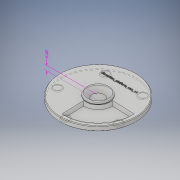
# Autodesk Inventor part: dissection_platform_v01
Saved by Autodesk Inventor 2019 (Build 230136000, 136)
## iProperties
Created: 2018-12-14
Part Number: dissection_platform_v01
Material: Generic
Document SubType Name: Modeling
Designer: Wilson Lab
Density: 1 g/cm^3
Appearance: Default
Author: Wilson Lab
Autodesk Inventor part; units mm, degrees
ref_plane "YZ Plane" through (0, 0, 0) normal (1, 0, 0) x (0, 1, 0)
ref_plane "XZ Plane" through (0, 0, 0) normal (0, 1, 0) x (-1, 0, 0)
ref_plane "XY Plane" through (0, 0, 0) normal (0, 0, 1) x (1, 0, 0)
sketch "Base Material Sketch" plane through (0, 0, 0) normal (0, 1, 0) x (-1, 0, 0)
  circle A0 centre (0, 0) radius 32.5
  dimension "d0" = 65
  constraints: 1 centre point, 1 coincident
  measures "d0" diameter of A0
extrude "Base Material Extrusion" add sketch "Base Material Sketch" along normal blind 4
sketch "Magnet Recess" plane through (0, 0, 0) normal (0, -1, 0) x (1, 0, 0)
  circle A0 centre (0, 0) radius 32.5 projected
  circle A1 centre (0, 27.5) radius 3.25
  line L0 (0, 0) -> (0, 32.5) construction
  circle A2 centre (0, 0) radius 32.5 construction
  circle A3 centre (-26.1541, 8.498) radius 3.25
  circle A4 centre (-16.1641, -22.248) radius 3.25
  circle A5 centre (16.1641, -22.248) radius 3.25
  circle A6 centre (26.1541, 8.498) radius 3.25
  dimension "d3" = 6.5
  dimension "d4" = 5
  dimension "d7" = 360
  constraints: 5 centre point, 2 end point, 1 point on line, 1 vertical, 1 vertical alignment, 12 other
  measures "d3" diameter of A1
  measures "d4" distance of A1.centre L0.end
extrude "Bottom Magnet Recess" cut sketch "Magnet Recess" against normal blind 1 contours A1 | A3 | A4 | A5 | A6
sketch "Central Well" plane through (0, 4, 0) normal (0, 1, 0) x (1, 0, 0)
  circle A0 centre (0, 0) radius 32.5 construction
  circle A1 centre (0, 0) radius 5
  dimension "d12" = 10
  constraints: 1 centre point, 1 coincident
  measures "d12" diameter of A1
extrude "Well Recess" cut sketch "Central Well" against normal blind 2
sketch "Sketch6" plane through (0, 4, 0) normal (0, 1, 0) x (1, 0, 0)
  circle A0 centre (0, 0) radius 9
  circle A1 centre (0, 0) radius 10
  dimension "d22" = 18
  dimension "d23" = 20
  constraints: 2 centre point, 2 coincident
  measures "d22" diameter of A0
  measures "d23" diameter of A1
extrude "Well Wall" add sketch "Sketch6" along normal blind 2
sketch "kimwipe recess sketch" plane through (0, 4, 0) normal (0, 1, 0) x (1, 0, 0)
  circle A0 centre (0, 0) radius 32.5 construction
  circle A1 centre (0, 0) radius 10 construction
  circle A2 centre (0, 0) radius 5 construction
  arc A3 (0, -12.5) -> (12.5, 0) centre (0, 0) ccw
  circle A4 centre (0, 0) radius 32.5 construction
  line L0 (0, 0) -> (-27.5, 0) construction
  line L1 (0, 0) -> (27.5, 0) construction
  line L2 (0, 0) -> (0, -27.5) construction
  line L3 (12.5, 0) -> (27.495, -0.5236)
  line L4 (0, -12.5) -> (0.5236, -27.495)
  arc A5 (0.5236, -27.495) -> (27.495, -0.5236) centre (0, 0) ccw
  dimension "d31" = 2.5
  dimension "d34" = 2
  dimension "d35" = 2
  dimension "d36" = 27.5
  constraints: 10 end point, 4 point on circle, 3 coincident, 2 centre point, 2 horizontal, 2 point on line, 1 perpendicular
  measures "d31" radial gap between concentric circles of A3 A1
  measures "d34" angle of L1 L3
  measures "d35" angle of L4 L2
  measures "d36" radius of A5
chamfer "Well Chamfer" distance 2 angle 45 2 edges at (-5, 4, 0) (-9, 4, 0)
fillet "Well Wall Fillet" radius 2 1 edges at (-10, 6, 0)
extrude "kimwipe recess" cut sketch "kimwipe recess sketch" against normal blind 2
chamfer "Kimwipe recess chamfer" distance 2 angle 45 4 edges at (0.2618, 4, 19.9975) (8.8388, 4, 8.8388) (19.9975, 4, 0.2618) (19.4454, 4, 19.4454)
fillet "Aesthetic Filet" radius 0.5 7 edges at (12.9141, 0, -22.248) (-19.4141, 0, -22.248) (-29.4041, 0, 8.498) (-3.25, 0, 27.5) (22.9041, 0, 8.498) (32.5, 0, 0) (32.5, 4, 0)
sketch "Sketch8" plane through (0, 4, 0) normal (0, 1, 0) x (1, 0, 0)
  line L0 (-6.854, 19.3116) -> (6.854, 19.3116) construction
  line L1 (6.854, 19.3116) -> (6.854, 17.5) construction
  line L2 (6.854, 17.5) -> (-6.854, 17.5) construction
  line L3 (-6.854, 17.5) -> (-6.854, 19.3116) construction
  circle A0 centre (0, 0) radius 17.5
  line L4 (-6.854, 17.5) -> (6.854, 17.5)
  line L5 (0, 0) -> (0, 17.5)
  line L6 (-14.128, 17.7085) -> (-14.3555, 17.7085)
  line L7 (-14.3555, 17.7085) -> (-14.3555, 17.8457)
  spline S0 degree 2 poles (-14.3555, 17.8457) (-14.408, 17.8019) (-14.4853, 17.7436) (-14.5378, 17.7188) knots 0 0 0 1 2 2 2
  spline S1 degree 2 poles (-14.5378, 17.7188) (-14.586, 17.6954) (-14.6895, 17.6706) (-14.7581, 17.6706) knots 0 0 0 1 2 2 2
  spline S2 degree 2 poles (-14.7581, 17.6706) (-14.869, 17.6706) (-15.0557, 17.7625) (-15.1213, 17.8515) knots 0 0 0 1 2 2 2
  spline S3 degree 2 poles (-15.1213, 17.8515) (-15.187, 17.9405) (-15.2599, 18.203) (-15.2599, 18.3737) knots 0 0 0 1 2 2 2
  spline S4 degree 2 poles (-15.2599, 18.3737) (-15.2599, 18.5517) (-15.168, 18.8113) (-15.0878, 18.909) knots 0 0 0 1 2 2 2
  spline S5 degree 2 poles (-15.0878, 18.909) (-15.0134, 18.9966) (-14.8048, 19.0972) (-14.6895, 19.0972) knots 0 0 0 1 2 2 2
  spline S6 degree 2 poles (-14.6895, 19.0972) (-14.5889, 19.0972) (-14.4387, 19.052) (-14.3555, 19.0053) knots 0 0 0 1 2 2 2
  line L8 (-14.3555, 19.0053) -> (-14.3555, 19.5888)
  line L9 (-14.3555, 19.5888) -> (-14.128, 19.5888)
  line L10 (-14.128, 19.5888) -> (-14.128, 17.7085)
  line L11 (-14.3555, 18.0368) -> (-14.3555, 18.8171)
  spline S7 degree 2 poles (-14.3555, 18.8171) (-14.4401, 18.858) (-14.5743, 18.8886) (-14.6516, 18.8886) knots 0 0 0 1 2 2 2
  spline S8 degree 2 poles (-14.6516, 18.8886) (-14.8267, 18.8886) (-15.025, 18.6261) (-15.025, 18.3781) knots 0 0 0 1 2 2 2
  spline S9 degree 2 poles (-15.025, 18.3781) (-15.025, 18.1389) (-14.8733, 17.8865) (-14.7056, 17.8865) knots 0 0 0 1 2 2 2
  spline S10 degree 2 poles (-14.7056, 17.8865) (-14.6166, 17.8865) (-14.4357, 17.9682) (-14.3555, 18.0368) knots 0 0 0 1 2 2 2
  line L12 (-13.5664, 17.7085) -> (-13.7939, 17.7085)
  line L13 (-13.7939, 17.7085) -> (-13.7939, 19.0593)
  line L14 (-13.7939, 19.0593) -> (-13.5664, 19.0593)
  line L15 (-13.5664, 19.0593) -> (-13.5664, 17.7085)
  line L16 (-13.5503, 19.2839) -> (-13.8085, 19.2839)
  line L17 (-13.8085, 19.2839) -> (-13.8085, 19.5202)
  line L18 (-13.8085, 19.5202) -> (-13.5503, 19.5202)
  line L19 (-13.5503, 19.5202) -> (-13.5503, 19.2839)
  spline S11 degree 2 poles (-12.8677, 17.6765) (-13.0033, 17.6765) (-13.2382, 17.7494) (-13.3155, 17.7902) knots 0 0 0 1 2 2 2
  line L20 (-13.3155, 17.7902) -> (-13.3155, 18.0455)
  line L21 (-13.3155, 18.0455) -> (-13.3038, 18.0455)
  spline S12 degree 2 poles (-13.3038, 18.0455) (-13.2746, 18.0222) (-13.1959, 17.9667) (-13.1302, 17.9361) knots 0 0 0 1 2 2 2
  spline S13 degree 2 poles (-13.1302, 17.9361) (-13.0733, 17.9084) (-12.9333, 17.8675) (-12.8589, 17.8675) knots 0 0 0 1 2 2 2
  spline S14 degree 2 poles (-12.8589, 17.8675) (-12.8049, 17.8675) (-12.681, 17.8923) (-12.6518, 17.9128) knots 0 0 0 1 2 2 2
  spline S15 degree 2 poles (-12.6518, 17.9128) (-12.6095, 17.9405) (-12.5716, 18.0032) (-12.5716, 18.0674) knots 0 0 0 1 2 2 2
  spline S16 degree 2 poles (-12.5716, 18.0674) (-12.5716, 18.1476) (-12.6591, 18.2308) (-12.7714, 18.2585) knots 0 0 0 1 2 2 2
  spline S17 degree 2 poles (-12.7714, 18.2585) (-12.8152, 18.2687) (-12.9552, 18.2979) (-13.015, 18.3139) knots 0 0 0 1 2 2 2
  spline S18 degree 2 poles (-13.015, 18.3139) (-13.1696, 18.3591) (-13.3096, 18.5458) (-13.3096, 18.6786) knots 0 0 0 1 2 2 2
  spline S19 degree 2 poles (-13.3096, 18.6786) (-13.3096, 18.8624) (-13.034, 19.0914) (-12.8064, 19.0914) knots 0 0 0 1 2 2 2
  spline S20 degree 2 poles (-12.8064, 19.0914) (-12.6941, 19.0914) (-12.4665, 19.0359) (-12.3892, 18.9936) knots 0 0 0 1 2 2 2
  line L22 (-12.3892, 18.9936) -> (-12.3892, 18.75)
  line L23 (-12.3892, 18.75) -> (-12.4009, 18.75)
  spline S21 degree 2 poles (-12.4009, 18.75) (-12.4884, 18.8201) (-12.7014, 18.9003) (-12.8108, 18.9003) knots 0 0 0 1 2 2 2
  spline S22 degree 2 poles (-12.8108, 18.9003) (-12.9231, 18.9003) (-13.0777, 18.8055) (-13.0777, 18.7107) knots 0 0 0 1 2 2 2
  spline S23 degree 2 poles (-13.0777, 18.7107) (-13.0777, 18.6246) (-12.9858, 18.5415) (-12.8837, 18.5152) knots 0 0 0 1 2 2 2
  spline S24 degree 2 poles (-12.8837, 18.5152) (-12.8341, 18.5021) (-12.7087, 18.4758) (-12.6401, 18.4598) knots 0 0 0 1 2 2 2
  spline S25 degree 2 poles (-12.6401, 18.4598) (-12.4913, 18.4218) (-12.3396, 18.2483) (-12.3396, 18.098) knots 0 0 0 1 2 2 2
  spline S26 degree 2 poles (-12.3396, 18.098) (-12.3396, 18.0105) (-12.4082, 17.8559) (-12.4753, 17.799) knots 0 0 0 1 2 2 2
  spline S27 degree 2 poles (-12.4753, 17.799) (-12.5468, 17.7392) (-12.7291, 17.6765) (-12.8677, 17.6765) knots 0 0 0 1 2 2 2
  spline S28 degree 2 poles (-11.7635, 17.6765) (-11.8991, 17.6765) (-12.134, 17.7494) (-12.2113, 17.7902) knots 0 0 0 1 2 2 2
  line L24 (-12.2113, 17.7902) -> (-12.2113, 18.0455)
  line L25 (-12.2113, 18.0455) -> (-12.1996, 18.0455)
  spline S29 degree 2 poles (-12.1996, 18.0455) (-12.1704, 18.0222) (-12.0917, 17.9667) (-12.026, 17.9361) knots 0 0 0 1 2 2 2
  spline S30 degree 2 poles (-12.026, 17.9361) (-11.9691, 17.9084) (-11.8291, 17.8675) (-11.7547, 17.8675) knots 0 0 0 1 2 2 2
  spline S31 degree 2 poles (-11.7547, 17.8675) (-11.7007, 17.8675) (-11.5767, 17.8923) (-11.5476, 17.9128) knots 0 0 0 1 2 2 2
  spline S32 degree 2 poles (-11.5476, 17.9128) (-11.5053, 17.9405) (-11.4673, 18.0032) (-11.4673, 18.0674) knots 0 0 0 1 2 2 2
  spline S33 degree 2 poles (-11.4673, 18.0674) (-11.4673, 18.1476) (-11.5549, 18.2308) (-11.6672, 18.2585) knots 0 0 0 1 2 2 2
  spline S34 degree 2 poles (-11.6672, 18.2585) (-11.7109, 18.2687) (-11.851, 18.2979) (-11.9108, 18.3139) knots 0 0 0 1 2 2 2
  spline S35 degree 2 poles (-11.9108, 18.3139) (-12.0654, 18.3591) (-12.2054, 18.5458) (-12.2054, 18.6786) knots 0 0 0 1 2 2 2
  spline S36 degree 2 poles (-12.2054, 18.6786) (-12.2054, 18.8624) (-11.9297, 19.0914) (-11.7022, 19.0914) knots 0 0 0 1 2 2 2
  spline S37 degree 2 poles (-11.7022, 19.0914) (-11.5899, 19.0914) (-11.3623, 19.0359) (-11.285, 18.9936) knots 0 0 0 1 2 2 2
  line L26 (-11.285, 18.9936) -> (-11.285, 18.75)
  line L27 (-11.285, 18.75) -> (-11.2967, 18.75)
  spline S38 degree 2 poles (-11.2967, 18.75) (-11.3842, 18.8201) (-11.5972, 18.9003) (-11.7066, 18.9003) knots 0 0 0 1 2 2 2
  spline S39 degree 2 poles (-11.7066, 18.9003) (-11.8189, 18.9003) (-11.9735, 18.8055) (-11.9735, 18.7107) knots 0 0 0 1 2 2 2
  spline S40 degree 2 poles (-11.9735, 18.7107) (-11.9735, 18.6246) (-11.8816, 18.5415) (-11.7795, 18.5152) knots 0 0 0 1 2 2 2
  spline S41 degree 2 poles (-11.7795, 18.5152) (-11.7299, 18.5021) (-11.6045, 18.4758) (-11.5359, 18.4598) knots 0 0 0 1 2 2 2
  spline S42 degree 2 poles (-11.5359, 18.4598) (-11.3871, 18.4218) (-11.2354, 18.2483) (-11.2354, 18.098) knots 0 0 0 1 2 2 2
  spline S43 degree 2 poles (-11.2354, 18.098) (-11.2354, 18.0105) (-11.304, 17.8559) (-11.3711, 17.799) knots 0 0 0 1 2 2 2
  spline S44 degree 2 poles (-11.3711, 17.799) (-11.4425, 17.7392) (-11.6249, 17.6765) (-11.7635, 17.6765) knots 0 0 0 1 2 2 2
  spline S45 degree 2 poles (-10.4375, 17.6779) (-10.7613, 17.6779) (-11.1173, 18.0411) (-11.1173, 18.3766) knots 0 0 0 1 2 2 2
  spline S46 degree 2 poles (-11.1173, 18.3766) (-11.1173, 18.7063) (-10.7716, 19.0972) (-10.4929, 19.0972) knots 0 0 0 1 2 2 2
  spline S47 degree 2 poles (-10.4929, 19.0972) (-10.3675, 19.0972) (-10.1735, 19.0243) (-10.102, 18.947) knots 0 0 0 1 2 2 2
  spline S48 degree 2 poles (-10.102, 18.947) (-10.0291, 18.8697) (-9.9518, 18.6465) (-9.9518, 18.4846) knots 0 0 0 1 2 2 2
  line L28 (-9.9518, 18.4846) -> (-9.9518, 18.3606)
  line L29 (-9.9518, 18.3606) -> (-10.8868, 18.3606)
  spline S49 degree 2 poles (-10.8868, 18.3606) (-10.8868, 18.1257) (-10.6505, 17.8763) (-10.4404, 17.8763) knots 0 0 0 1 2 2 2
  spline S50 degree 2 poles (-10.4404, 17.8763) (-10.366, 17.8763) (-10.2216, 17.9098) (-10.1633, 17.9361) knots 0 0 0 1 2 2 2
  spline S51 degree 2 poles (-10.1633, 17.9361) (-10.102, 17.9653) (-10.0174, 18.0163) (-9.9897, 18.0397) knots 0 0 0 1 2 2 2
  line L30 (-9.9897, 18.0397) -> (-9.9766, 18.0397)
  line L31 (-9.9766, 18.0397) -> (-9.9766, 17.7917)
  spline S52 degree 2 poles (-9.9766, 17.7917) (-10.016, 17.7756) (-10.1356, 17.729) (-10.1823, 17.7158) knots 0 0 0 1 2 2 2
  spline S53 degree 2 poles (-10.1823, 17.7158) (-10.2479, 17.6969) (-10.3558, 17.6779) (-10.4375, 17.6779) knots 0 0 0 1 2 2 2
  spline S54 degree 2 poles (-10.1735, 18.5342) (-10.1764, 18.6261) (-10.2143, 18.7603) (-10.2508, 18.8055) knots 0 0 0 1 2 2 2
  spline S55 degree 2 poles (-10.2508, 18.8055) (-10.2902, 18.8565) (-10.4142, 18.9105) (-10.5061, 18.9105) knots 0 0 0 1 2 2 2
  spline S56 degree 2 poles (-10.5061, 18.9105) (-10.5965, 18.9105) (-10.7234, 18.8565) (-10.7759, 18.804) knots 0 0 0 1 2 2 2
  spline S57 degree 2 poles (-10.7759, 18.804) (-10.827, 18.75) (-10.8795, 18.6202) (-10.8868, 18.5342) knots 0 0 0 1 2 2 2
  line L32 (-10.8868, 18.5342) -> (-10.1735, 18.5342)
  spline S58 degree 2 poles (-9.1845, 17.6779) (-9.3246, 17.6779) (-9.5565, 17.764) (-9.6396, 17.8515) knots 0 0 0 1 2 2 2
  spline S59 degree 2 poles (-9.6396, 17.8515) (-9.7228, 17.9376) (-9.8147, 18.203) (-9.8147, 18.381) knots 0 0 0 1 2 2 2
  spline S60 degree 2 poles (-9.8147, 18.381) (-9.8147, 18.559) (-9.7199, 18.8186) (-9.6396, 18.9061) knots 0 0 0 1 2 2 2
  spline S61 degree 2 poles (-9.6396, 18.9061) (-9.5594, 18.9951) (-9.3216, 19.0899) (-9.1845, 19.0899) knots 0 0 0 1 2 2 2
  spline S62 degree 2 poles (-9.1845, 19.0899) (-9.0737, 19.0899) (-8.8665, 19.0272) (-8.7863, 18.9863) knots 0 0 0 1 2 2 2
  line L33 (-8.7863, 18.9863) -> (-8.7863, 18.7311)
  line L34 (-8.7863, 18.7311) -> (-8.7994, 18.7311)
  spline S63 degree 2 poles (-8.7994, 18.7311) (-8.8242, 18.7515) (-8.9001, 18.804) (-8.9541, 18.8317) knots 0 0 0 1 2 2 2
  spline S64 degree 2 poles (-8.9541, 18.8317) (-9.0022, 18.8551) (-9.1306, 18.8915) (-9.1889, 18.8915) knots 0 0 0 1 2 2 2
  spline S65 degree 2 poles (-9.1889, 18.8915) (-9.3654, 18.8915) (-9.5798, 18.6246) (-9.5798, 18.381) knots 0 0 0 1 2 2 2
  spline S66 degree 2 poles (-9.5798, 18.381) (-9.5798, 18.1432) (-9.3727, 17.8763) (-9.1889, 17.8763) knots 0 0 0 1 2 2 2
  spline S67 degree 2 poles (-9.1889, 17.8763) (-9.078, 17.8763) (-8.8767, 17.9682) (-8.7994, 18.0397) knots 0 0 0 1 2 2 2
  line L35 (-8.7994, 18.0397) -> (-8.7863, 18.0397)
  line L36 (-8.7863, 18.0397) -> (-8.7863, 17.7844)
  spline S68 degree 2 poles (-8.7863, 17.7844) (-8.8199, 17.7684) (-8.922, 17.7231) (-8.9628, 17.7129) knots 0 0 0 1 2 2 2
  spline S69 degree 2 poles (-8.9628, 17.7129) (-9.0212, 17.6954) (-9.113, 17.6779) (-9.1845, 17.6779) knots 0 0 0 1 2 2 2
  spline S70 degree 2 poles (-8.1707, 17.6823) (-8.356, 17.6823) (-8.5646, 17.8938) (-8.5646, 18.1228) knots 0 0 0 1 2 2 2
  line L37 (-8.5646, 18.1228) -> (-8.5646, 18.8711)
  line L38 (-8.5646, 18.8711) -> (-8.7177, 18.8711)
  line L39 (-8.7177, 18.8711) -> (-8.7177, 19.0593)
  line L40 (-8.7177, 19.0593) -> (-8.5646, 19.0593)
  line L41 (-8.5646, 19.0593) -> (-8.5646, 19.4473)
  line L42 (-8.5646, 19.4473) -> (-8.337, 19.4473)
  line L43 (-8.337, 19.4473) -> (-8.337, 19.0593)
  line L44 (-8.337, 19.0593) -> (-7.9184, 19.0593)
  line L45 (-7.9184, 19.0593) -> (-7.9184, 18.8711)
  line L46 (-7.9184, 18.8711) -> (-8.337, 18.8711)
  line L47 (-8.337, 18.8711) -> (-8.337, 18.2278)
  spline S71 degree 2 poles (-8.337, 18.2278) (-8.337, 18.1257) (-8.3297, 18.0134) (-8.3049, 17.9653) knots 0 0 0 1 2 2 2
  spline S72 degree 2 poles (-8.3049, 17.9653) (-8.2845, 17.923) (-8.1926, 17.8807) (-8.1139, 17.8807) knots 0 0 0 1 2 2 2
  spline S73 degree 2 poles (-8.1139, 17.8807) (-8.0584, 17.8807) (-7.9549, 17.9142) (-7.9315, 17.9244) knots 0 0 0 1 2 2 2
  line L48 (-7.9315, 17.9244) -> (-7.9184, 17.9244)
  line L49 (-7.9184, 17.9244) -> (-7.9184, 17.7202)
  spline S74 degree 2 poles (-7.9184, 17.7202) (-7.9826, 17.7027) (-8.1139, 17.6823) (-8.1707, 17.6823) knots 0 0 0 1 2 2 2
  line L50 (-7.5187, 17.7085) -> (-7.7463, 17.7085)
  line L51 (-7.7463, 17.7085) -> (-7.7463, 19.0593)
  line L52 (-7.7463, 19.0593) -> (-7.5187, 19.0593)
  line L53 (-7.5187, 19.0593) -> (-7.5187, 17.7085)
  line L54 (-7.5027, 19.2839) -> (-7.7609, 19.2839)
  line L55 (-7.7609, 19.2839) -> (-7.7609, 19.5202)
  line L56 (-7.7609, 19.5202) -> (-7.5027, 19.5202)
  line L57 (-7.5027, 19.5202) -> (-7.5027, 19.2839)
  spline S75 degree 2 poles (-6.0746, 18.3839) (-6.0746, 18.0426) (-6.4028, 17.6706) (-6.6771, 17.6706) knots 0 0 0 1 2 2 2
  spline S76 degree 2 poles (-6.6771, 17.6706) (-6.9586, 17.6706) (-7.281, 18.0543) (-7.281, 18.3839) knots 0 0 0 1 2 2 2
  spline S77 degree 2 poles (-7.281, 18.3839) (-7.281, 18.7223) (-6.9484, 19.0972) (-6.6771, 19.0972) knots 0 0 0 1 2 2 2
  spline S78 degree 2 poles (-6.6771, 19.0972) (-6.4028, 19.0972) (-6.0746, 18.7238) (-6.0746, 18.3839) knots 0 0 0 1 2 2 2
  spline S79 degree 2 poles (-6.3095, 18.3839) (-6.3095, 18.6465) (-6.5006, 18.9017) (-6.6771, 18.9017) knots 0 0 0 1 2 2 2
  spline S80 degree 2 poles (-6.6771, 18.9017) (-6.8536, 18.9017) (-7.0461, 18.6465) (-7.0461, 18.3839) knots 0 0 0 1 2 2 2
  spline S81 degree 2 poles (-7.0461, 18.3839) (-7.0461, 18.1286) (-6.8536, 17.8661) (-6.6771, 17.8661) knots 0 0 0 1 2 2 2
  spline S82 degree 2 poles (-6.6771, 17.8661) (-6.502, 17.8661) (-6.3095, 18.1243) (-6.3095, 18.3839) knots 0 0 0 1 2 2 2
  line L58 (-4.7808, 17.7085) -> (-5.0083, 17.7085)
  line L59 (-5.0083, 17.7085) -> (-5.0083, 18.4787)
  spline S83 degree 2 poles (-5.0083, 18.4787) (-5.0083, 18.5721) (-5.0259, 18.7325) (-5.0521, 18.7807) knots 0 0 0 1 2 2 2
  spline S84 degree 2 poles (-5.0521, 18.7807) (-5.0798, 18.8317) (-5.179, 18.8813) (-5.2636, 18.8813) knots 0 0 0 1 2 2 2
  spline S85 degree 2 poles (-5.2636, 18.8813) (-5.3482, 18.8813) (-5.5276, 18.7909) (-5.6137, 18.718) knots 0 0 0 1 2 2 2
  line L60 (-5.6137, 18.718) -> (-5.6137, 17.7085)
  line L61 (-5.6137, 17.7085) -> (-5.8412, 17.7085)
  line L62 (-5.8412, 17.7085) -> (-5.8412, 19.0593)
  line L63 (-5.8412, 19.0593) -> (-5.6137, 19.0593)
  line L64 (-5.6137, 19.0593) -> (-5.6137, 18.909)
  spline S86 degree 2 poles (-5.6137, 18.909) (-5.5116, 19.0009) (-5.3147, 19.0972) (-5.2038, 19.0972) knots 0 0 0 1 2 2 2
  spline S87 degree 2 poles (-5.2038, 19.0972) (-5.0054, 19.0972) (-4.7808, 18.8346) (-4.7808, 18.5852) knots 0 0 0 1 2 2 2
  line L65 (-4.7808, 18.5852) -> (-4.7808, 17.7085)
  line L66 (-3.2565, 17.3468) -> (-4.6451, 17.3468)
  line L67 (-4.6451, 17.3468) -> (-4.6451, 17.5029)
  line L68 (-4.6451, 17.5029) -> (-3.2565, 17.5029)
  line L69 (-3.2565, 17.5029) -> (-3.2565, 17.3468)
  spline S88 degree 2 poles (-1.9787, 18.4204) (-1.9787, 18.082) (-2.3011, 17.6823) (-2.5476, 17.6823) knots 0 0 0 1 2 2 2
  spline S89 degree 2 poles (-2.5476, 17.6823) (-2.6482, 17.6823) (-2.8028, 17.729) (-2.8831, 17.7771) knots 0 0 0 1 2 2 2
  line L70 (-2.8831, 17.7771) -> (-2.8831, 17.2111)
  line L71 (-2.8831, 17.2111) -> (-3.1106, 17.2111)
  line L72 (-3.1106, 17.2111) -> (-3.1106, 19.0593)
  line L73 (-3.1106, 19.0593) -> (-2.8831, 19.0593)
  line L74 (-2.8831, 19.0593) -> (-2.8831, 18.9178)
  spline S90 degree 2 poles (-2.8831, 18.9178) (-2.7985, 18.9951) (-2.5913, 19.0972) (-2.4703, 19.0972) knots 0 0 0 1 2 2 2
  spline S91 degree 2 poles (-2.4703, 19.0972) (-2.2383, 19.0972) (-1.9787, 18.7296) (-1.9787, 18.4204) knots 0 0 0 1 2 2 2
  spline S92 degree 2 poles (-2.2135, 18.3941) (-2.2135, 18.6261) (-2.3609, 18.8813) (-2.5257, 18.8813) knots 0 0 0 1 2 2 2
  spline S93 degree 2 poles (-2.5257, 18.8813) (-2.622, 18.8813) (-2.8028, 18.7953) (-2.8831, 18.7282) knots 0 0 0 1 2 2 2
  line L75 (-2.8831, 18.7282) -> (-2.8831, 17.9609)
  spline S94 degree 2 poles (-2.8831, 17.9609) (-2.7941, 17.9186) (-2.6672, 17.8865) (-2.5855, 17.8865) knots 0 0 0 1 2 2 2
  spline S95 degree 2 poles (-2.5855, 17.8865) (-2.409, 17.8865) (-2.2135, 18.1462) (-2.2135, 18.3941) knots 0 0 0 1 2 2 2
  line L76 (-1.5105, 17.7085) -> (-1.738, 17.7085)
  line L77 (-1.738, 17.7085) -> (-1.738, 19.5888)
  line L78 (-1.738, 19.5888) -> (-1.5105, 19.5888)
  line L79 (-1.5105, 19.5888) -> (-1.5105, 17.7085)
  spline S96 degree 2 poles (-0.4237, 17.8515) (-0.4515, 17.8311) (-0.5448, 17.7581) (-0.5886, 17.7363) knots 0 0 0 1 2 2 2
  spline S97 degree 2 poles (-0.5886, 17.7363) (-0.6484, 17.7042) (-0.7607, 17.6706) (-0.8628, 17.6706) knots 0 0 0 1 2 2 2
  spline S98 degree 2 poles (-0.8628, 17.6706) (-0.9459, 17.6706) (-1.0962, 17.7333) (-1.1531, 17.7902) knots 0 0 0 1 2 2 2
  spline S99 degree 2 poles (-1.1531, 17.7902) (-1.207, 17.8457) (-1.2727, 18.009) (-1.2727, 18.0995) knots 0 0 0 1 2 2 2
  spline S100 degree 2 poles (-1.2727, 18.0995) (-1.2727, 18.2395) (-1.1545, 18.4379) (-1.0262, 18.4948) knots 0 0 0 1 2 2 2
  spline S101 degree 2 poles (-1.0262, 18.4948) (-0.9124, 18.5473) (-0.6032, 18.5867) (-0.4237, 18.5969) knots 0 0 0 1 2 2 2
  line L80 (-0.4237, 18.5969) -> (-0.4237, 18.6406)
  spline S102 degree 2 poles (-0.4237, 18.6406) (-0.4237, 18.7194) (-0.4719, 18.8171) (-0.5156, 18.8449) knots 0 0 0 1 2 2 2
  spline S103 degree 2 poles (-0.5156, 18.8449) (-0.5594, 18.8726) (-0.6848, 18.8901) (-0.7519, 18.8901) knots 0 0 0 1 2 2 2
  spline S104 degree 2 poles (-0.7519, 18.8901) (-0.8307, 18.8901) (-1.0437, 18.8434) (-1.1502, 18.7982) knots 0 0 0 1 2 2 2
  line L81 (-1.1502, 18.7982) -> (-1.1633, 18.7982)
  line L82 (-1.1633, 18.7982) -> (-1.1633, 19.0301)
  spline S105 degree 2 poles (-1.1633, 19.0301) (-1.1006, 19.0476) (-0.8657, 19.0914) (-0.7505, 19.0914) knots 0 0 0 1 2 2 2
  spline S106 degree 2 poles (-0.7505, 19.0914) (-0.6105, 19.0914) (-0.4194, 19.0476) (-0.3435, 18.9907) knots 0 0 0 1 2 2 2
  spline S107 degree 2 poles (-0.3435, 18.9907) (-0.2691, 18.9353) (-0.1962, 18.7588) (-0.1962, 18.6319) knots 0 0 0 1 2 2 2
  line L83 (-0.1962, 18.6319) -> (-0.1962, 17.7085)
  line L84 (-0.1962, 17.7085) -> (-0.4237, 17.7085)
  line L85 (-0.4237, 17.7085) -> (-0.4237, 17.8515)
  line L86 (-0.4237, 18.0411) -> (-0.4237, 18.416)
  spline S108 degree 2 poles (-0.4237, 18.416) (-0.5054, 18.4087) (-0.7519, 18.3839) (-0.8293, 18.3606) knots 0 0 0 1 2 2 2
  spline S109 degree 2 poles (-0.8293, 18.3606) (-0.9197, 18.3329) (-1.0378, 18.2176) (-1.0378, 18.1155) knots 0 0 0 1 2 2 2
  spline S110 degree 2 poles (-1.0378, 18.1155) (-1.0378, 17.9988) (-0.9066, 17.8807) (-0.7811, 17.8807) knots 0 0 0 1 2 2 2
  spline S111 degree 2 poles (-0.7811, 17.8807) (-0.6746, 17.8807) (-0.4996, 17.9726) (-0.4237, 18.0411) knots 0 0 0 1 2 2 2
  spline S112 degree 2 poles (0.5317, 17.6823) (0.3464, 17.6823) (0.1378, 17.8938) (0.1378, 18.1228) knots 0 0 0 1 2 2 2
  line L87 (0.1378, 18.1228) -> (0.1378, 18.8711)
  line L88 (0.1378, 18.8711) -> (-0.0153, 18.8711)
  line L89 (-0.0153, 18.8711) -> (-0.0153, 19.0593)
  line L90 (-0.0153, 19.0593) -> (0.1378, 19.0593)
  line L91 (0.1378, 19.0593) -> (0.1378, 19.4473)
  line L92 (0.1378, 19.4473) -> (0.3654, 19.4473)
  line L93 (0.3654, 19.4473) -> (0.3654, 19.0593)
  line L94 (0.3654, 19.0593) -> (0.784, 19.0593)
  line L95 (0.784, 19.0593) -> (0.784, 18.8711)
  line L96 (0.784, 18.8711) -> (0.3654, 18.8711)
  line L97 (0.3654, 18.8711) -> (0.3654, 18.2278)
  spline S113 degree 2 poles (0.3654, 18.2278) (0.3654, 18.1257) (0.3727, 18.0134) (0.3975, 17.9653) knots 0 0 0 1 2 2 2
  spline S114 degree 2 poles (0.3975, 17.9653) (0.4179, 17.923) (0.5098, 17.8807) (0.5886, 17.8807) knots 0 0 0 1 2 2 2
  spline S115 degree 2 poles (0.5886, 17.8807) (0.644, 17.8807) (0.7476, 17.9142) (0.7709, 17.9244) knots 0 0 0 1 2 2 2
  line L98 (0.7709, 17.9244) -> (0.784, 17.9244)
  line L99 (0.784, 17.9244) -> (0.784, 17.7202)
  spline S116 degree 2 poles (0.784, 17.7202) (0.7199, 17.7027) (0.5886, 17.6823) (0.5317, 17.6823) knots 0 0 0 1 2 2 2
  line L100 (1.6622, 19.37) -> (1.6505, 19.37)
  spline S117 degree 2 poles (1.6505, 19.37) (1.6199, 19.3816) (1.5061, 19.4021) (1.4609, 19.4021) knots 0 0 0 1 2 2 2
  spline S118 degree 2 poles (1.4609, 19.4021) (1.3179, 19.4021) (1.1954, 19.2737) (1.1954, 19.1045) knots 0 0 0 1 2 2 2
  line L101 (1.1954, 19.1045) -> (1.1954, 19.0593)
  line L102 (1.1954, 19.0593) -> (1.5717, 19.0593)
  line L103 (1.5717, 19.0593) -> (1.5717, 18.8711)
  line L104 (1.5717, 18.8711) -> (1.2027, 18.8711)
  line L105 (1.2027, 18.8711) -> (1.2027, 17.7085)
  line L106 (1.2027, 17.7085) -> (0.9751, 17.7085)
  line L107 (0.9751, 17.7085) -> (0.9751, 18.8711)
  line L108 (0.9751, 18.8711) -> (0.822, 18.8711)
  line L109 (0.822, 18.8711) -> (0.822, 19.0593)
  line L110 (0.822, 19.0593) -> (0.9751, 19.0593)
  line L111 (0.9751, 19.0593) -> (0.9751, 19.1045)
  spline S119 degree 2 poles (0.9751, 19.1045) (0.9751, 19.3466) (1.21, 19.6004) (1.4288, 19.6004) knots 0 0 0 1 2 2 2
  spline S120 degree 2 poles (1.4288, 19.6004) (1.4915, 19.6004) (1.6126, 19.5873) (1.6622, 19.5786) knots 0 0 0 1 2 2 2
  line L112 (1.6622, 19.5786) -> (1.6622, 19.37)
  spline S121 degree 2 poles (2.8495, 18.3839) (2.8495, 18.0426) (2.5213, 17.6706) (2.2471, 17.6706) knots 0 0 0 1 2 2 2
  spline S122 degree 2 poles (2.2471, 17.6706) (1.9656, 17.6706) (1.6432, 18.0543) (1.6432, 18.3839) knots 0 0 0 1 2 2 2
  spline S123 degree 2 poles (1.6432, 18.3839) (1.6432, 18.7223) (1.9758, 19.0972) (2.2471, 19.0972) knots 0 0 0 1 2 2 2
  spline S124 degree 2 poles (2.2471, 19.0972) (2.5213, 19.0972) (2.8495, 18.7238) (2.8495, 18.3839) knots 0 0 0 1 2 2 2
  spline S125 degree 2 poles (2.6147, 18.3839) (2.6147, 18.6465) (2.4236, 18.9017) (2.2471, 18.9017) knots 0 0 0 1 2 2 2
  spline S126 degree 2 poles (2.2471, 18.9017) (2.0706, 18.9017) (1.878, 18.6465) (1.878, 18.3839) knots 0 0 0 1 2 2 2
  spline S127 degree 2 poles (1.878, 18.3839) (1.878, 18.1286) (2.0706, 17.8661) (2.2471, 17.8661) knots 0 0 0 1 2 2 2
  spline S128 degree 2 poles (2.2471, 17.8661) (2.4221, 17.8661) (2.6147, 18.1243) (2.6147, 18.3839) knots 0 0 0 1 2 2 2
  line L113 (3.7991, 18.8157) -> (3.7874, 18.8157)
  spline S129 degree 2 poles (3.7874, 18.8157) (3.7612, 18.823) (3.7043, 18.8259) (3.6649, 18.8259) knots 0 0 0 1 2 2 2
  spline S130 degree 2 poles (3.6649, 18.8259) (3.573, 18.8259) (3.3921, 18.7457) (3.3105, 18.6669) knots 0 0 0 1 2 2 2
  line L114 (3.3105, 18.6669) -> (3.3105, 17.7085)
  line L115 (3.3105, 17.7085) -> (3.0829, 17.7085)
  line L116 (3.0829, 17.7085) -> (3.0829, 19.0593)
  line L117 (3.0829, 19.0593) -> (3.3105, 19.0593)
  line L118 (3.3105, 19.0593) -> (3.3105, 18.858)
  spline S131 degree 2 poles (3.3105, 18.858) (3.4344, 18.9688) (3.6197, 19.0593) (3.7072, 19.0593) knots 0 0 0 1 2 2 2
  spline S132 degree 2 poles (3.7072, 19.0593) (3.7422, 19.0593) (3.7772, 19.0564) (3.7991, 19.052) knots 0 0 0 1 2 2 2
  line L119 (3.7991, 19.052) -> (3.7991, 18.8157)
  line L120 (5.5072, 17.7085) -> (5.5072, 18.4904)
  spline S133 degree 2 poles (5.5072, 18.4904) (5.5072, 18.5838) (5.4926, 18.7427) (5.4693, 18.7865) knots 0 0 0 1 2 2 2
  spline S134 degree 2 poles (5.4693, 18.7865) (5.4459, 18.8346) (5.357, 18.8813) (5.2797, 18.8813) knots 0 0 0 1 2 2 2
  spline S135 degree 2 poles (5.2797, 18.8813) (5.2096, 18.8813) (5.0492, 18.7953) (4.9646, 18.7136) knots 0 0 0 1 2 2 2
  spline S136 degree 2 poles (4.9646, 18.7136) (4.966, 18.6932) (4.969, 18.6363) (4.969, 18.5983) knots 0 0 0 1 2 2 2
  line L121 (4.969, 18.5983) -> (4.969, 17.7085)
  line L122 (4.969, 17.7085) -> (4.7414, 17.7085)
  line L123 (4.7414, 17.7085) -> (4.7414, 18.4904)
  spline S137 degree 2 poles (4.7414, 18.4904) (4.7414, 18.5838) (4.7268, 18.7427) (4.7035, 18.7865) knots 0 0 0 1 2 2 2
  spline S138 degree 2 poles (4.7035, 18.7865) (4.6801, 18.8346) (4.5912, 18.8813) (4.5139, 18.8813) knots 0 0 0 1 2 2 2
  spline S139 degree 2 poles (4.5139, 18.8813) (4.4409, 18.8813) (4.279, 18.7894) (4.2032, 18.718) knots 0 0 0 1 2 2 2
  line L124 (4.2032, 18.718) -> (4.2032, 17.7085)
  line L125 (4.2032, 17.7085) -> (3.9756, 17.7085)
  line L126 (3.9756, 17.7085) -> (3.9756, 19.0593)
  line L127 (3.9756, 19.0593) -> (4.2032, 19.0593)
  line L128 (4.2032, 19.0593) -> (4.2032, 18.9105)
  spline S140 degree 2 poles (4.2032, 18.9105) (4.2921, 18.9995) (4.4672, 19.0972) (4.5722, 19.0972) knots 0 0 0 1 2 2 2
  spline S141 degree 2 poles (4.5722, 19.0972) (4.6918, 19.0972) (4.8771, 18.9878) (4.9252, 18.8638) knots 0 0 0 1 2 2 2
  spline S142 degree 2 poles (4.9252, 18.8638) (5.0288, 18.9791) (5.2242, 19.0972) (5.338, 19.0972) knots 0 0 0 1 2 2 2
  spline S143 degree 2 poles (5.338, 19.0972) (5.4255, 19.0972) (5.5685, 19.0432) (5.621, 18.982) knots 0 0 0 1 2 2 2
  spline S144 degree 2 poles (5.621, 18.982) (5.675, 18.9207) (5.7348, 18.7369) (5.7348, 18.5983) knots 0 0 0 1 2 2 2
  line L129 (5.7348, 18.5983) -> (5.7348, 17.7085)
  line L130 (5.7348, 17.7085) -> (5.5072, 17.7085)
  line L131 (7.2591, 17.3468) -> (5.8704, 17.3468)
  line L132 (5.8704, 17.3468) -> (5.8704, 17.5029)
  line L133 (5.8704, 17.5029) -> (7.2591, 17.5029)
  line L134 (7.2591, 17.5029) -> (7.2591, 17.3468)
  line L135 (8.9365, 17.7085) -> (8.9365, 18.4904)
  spline S145 degree 2 poles (8.9365, 18.4904) (8.9365, 18.5838) (8.922, 18.7427) (8.8986, 18.7865) knots 0 0 0 1 2 2 2
  spline S146 degree 2 poles (8.8986, 18.7865) (8.8753, 18.8346) (8.7863, 18.8813) (8.709, 18.8813) knots 0 0 0 1 2 2 2
  spline S147 degree 2 poles (8.709, 18.8813) (8.639, 18.8813) (8.4785, 18.7953) (8.3939, 18.7136) knots 0 0 0 1 2 2 2
  spline S148 degree 2 poles (8.3939, 18.7136) (8.3954, 18.6932) (8.3983, 18.6363) (8.3983, 18.5983) knots 0 0 0 1 2 2 2
  line L136 (8.3983, 18.5983) -> (8.3983, 17.7085)
  line L137 (8.3983, 17.7085) -> (8.1707, 17.7085)
  line L138 (8.1707, 17.7085) -> (8.1707, 18.4904)
  spline S149 degree 2 poles (8.1707, 18.4904) (8.1707, 18.5838) (8.1562, 18.7427) (8.1328, 18.7865) knots 0 0 0 1 2 2 2
  spline S150 degree 2 poles (8.1328, 18.7865) (8.1095, 18.8346) (8.0205, 18.8813) (7.9432, 18.8813) knots 0 0 0 1 2 2 2
  spline S151 degree 2 poles (7.9432, 18.8813) (7.8703, 18.8813) (7.7083, 18.7894) (7.6325, 18.718) knots 0 0 0 1 2 2 2
  line L139 (7.6325, 18.718) -> (7.6325, 17.7085)
  line L140 (7.6325, 17.7085) -> (7.4049, 17.7085)
  line L141 (7.4049, 17.7085) -> (7.4049, 19.0593)
  line L142 (7.4049, 19.0593) -> (7.6325, 19.0593)
  line L143 (7.6325, 19.0593) -> (7.6325, 18.9105)
  spline S152 degree 2 poles (7.6325, 18.9105) (7.7215, 18.9995) (7.8965, 19.0972) (8.0015, 19.0972) knots 0 0 0 1 2 2 2
  spline S153 degree 2 poles (8.0015, 19.0972) (8.1212, 19.0972) (8.3064, 18.9878) (8.3545, 18.8638) knots 0 0 0 1 2 2 2
  spline S154 degree 2 poles (8.3545, 18.8638) (8.4581, 18.9791) (8.6536, 19.0972) (8.7673, 19.0972) knots 0 0 0 1 2 2 2
  spline S155 degree 2 poles (8.7673, 19.0972) (8.8549, 19.0972) (8.9978, 19.0432) (9.0503, 18.982) knots 0 0 0 1 2 2 2
  spline S156 degree 2 poles (9.0503, 18.982) (9.1043, 18.9207) (9.1641, 18.7369) (9.1641, 18.5983) knots 0 0 0 1 2 2 2
  line L144 (9.1641, 18.5983) -> (9.1641, 17.7085)
  line L145 (9.1641, 17.7085) -> (8.9365, 17.7085)
  line L146 (11.0152, 17.7085) -> (11.0152, 18.4904)
  spline S157 degree 2 poles (11.0152, 18.4904) (11.0152, 18.5838) (11.0006, 18.7427) (10.9772, 18.7865) knots 0 0 0 1 2 2 2
  spline S158 degree 2 poles (10.9772, 18.7865) (10.9539, 18.8346) (10.8649, 18.8813) (10.7876, 18.8813) knots 0 0 0 1 2 2 2
  spline S159 degree 2 poles (10.7876, 18.8813) (10.7176, 18.8813) (10.5571, 18.7953) (10.4725, 18.7136) knots 0 0 0 1 2 2 2
  spline S160 degree 2 poles (10.4725, 18.7136) (10.474, 18.6932) (10.4769, 18.6363) (10.4769, 18.5983) knots 0 0 0 1 2 2 2
  line L147 (10.4769, 18.5983) -> (10.4769, 17.7085)
  line L148 (10.4769, 17.7085) -> (10.2494, 17.7085)
  line L149 (10.2494, 17.7085) -> (10.2494, 18.4904)
  spline S161 degree 2 poles (10.2494, 18.4904) (10.2494, 18.5838) (10.2348, 18.7427) (10.2114, 18.7865) knots 0 0 0 1 2 2 2
  spline S162 degree 2 poles (10.2114, 18.7865) (10.1881, 18.8346) (10.0991, 18.8813) (10.0218, 18.8813) knots 0 0 0 1 2 2 2
  spline S163 degree 2 poles (10.0218, 18.8813) (9.9489, 18.8813) (9.787, 18.7894) (9.7111, 18.718) knots 0 0 0 1 2 2 2
  line L150 (9.7111, 18.718) -> (9.7111, 17.7085)
  line L151 (9.7111, 17.7085) -> (9.4836, 17.7085)
  line L152 (9.4836, 17.7085) -> (9.4836, 19.0593)
  line L153 (9.4836, 19.0593) -> (9.7111, 19.0593)
  line L154 (9.7111, 19.0593) -> (9.7111, 18.9105)
  spline S164 degree 2 poles (9.7111, 18.9105) (9.8001, 18.9995) (9.9751, 19.0972) (10.0801, 19.0972) knots 0 0 0 1 2 2 2
  spline S165 degree 2 poles (10.0801, 19.0972) (10.1998, 19.0972) (10.385, 18.9878) (10.4331, 18.8638) knots 0 0 0 1 2 2 2
  spline S166 degree 2 poles (10.4331, 18.8638) (10.5367, 18.9791) (10.7322, 19.0972) (10.8459, 19.0972) knots 0 0 0 1 2 2 2
  spline S167 degree 2 poles (10.8459, 19.0972) (10.9335, 19.0972) (11.0764, 19.0432) (11.1289, 18.982) knots 0 0 0 1 2 2 2
  spline S168 degree 2 poles (11.1289, 18.982) (11.1829, 18.9207) (11.2427, 18.7369) (11.2427, 18.5983) knots 0 0 0 1 2 2 2
  line L155 (11.2427, 18.5983) -> (11.2427, 17.7085)
  line L156 (11.2427, 17.7085) -> (11.0152, 17.7085)
  line L157 (12.767, 17.3468) -> (11.3784, 17.3468)
  line L158 (11.3784, 17.3468) -> (11.3784, 17.5029)
  line L159 (11.3784, 17.5029) -> (12.767, 17.5029)
  line L160 (12.767, 17.5029) -> (12.767, 17.3468)
  line L161 (13.9733, 19.0593) -> (13.4643, 17.7085)
  line L162 (13.4643, 17.7085) -> (13.26, 17.7085)
  line L163 (13.26, 17.7085) -> (12.7553, 19.0593)
  line L164 (12.7553, 19.0593) -> (13.0019, 19.0593)
  line L165 (13.0019, 19.0593) -> (13.3709, 18.0192)
  line L166 (13.3709, 18.0192) -> (13.737, 19.0593)
  line L167 (13.737, 19.0593) -> (13.9733, 19.0593)
  line L168 (15.1315, 17.7085) -> (14.2534, 17.7085)
  line L169 (14.2534, 17.7085) -> (14.2534, 17.8923)
  line L170 (14.2534, 17.8923) -> (14.5801, 17.8923)
  line L171 (14.5801, 17.8923) -> (14.5801, 19.0987)
  line L172 (14.5801, 19.0987) -> (14.2534, 19.0987)
  line L173 (14.2534, 19.0987) -> (14.2534, 19.2635)
  spline S169 degree 2 poles (14.2534, 19.2635) (14.4387, 19.2635) (14.6137, 19.3685) (14.6254, 19.5144) knots 0 0 0 1 2 2 2
  line L174 (14.6254, 19.5144) -> (14.8121, 19.5144)
  line L175 (14.8121, 19.5144) -> (14.8121, 17.8923)
  line L176 (14.8121, 17.8923) -> (15.1315, 17.8923)
  line L177 (15.1315, 17.8923) -> (15.1315, 17.7085)
  dimension "d46" = 35
  constraints: 4 end point, 2 midpoint, 1 coincident, 1 collinear, 1 vertical, 1 vertical alignment, 4 other
extrude "Extrusion7" cut sketch "Sketch8" against normal blind 0.35 contours L72 L4 L70 A0 | A0 L70 L71 L72 | L4 L72 L73 L74 S90 S91 S88 S89 L70 | L67 L68 L69 L4 | L4 L69 L66 L67 | L6 L7 S0 S1 S2 S3 S4 S5 S6 L8 L9 L10 | L12 L13 L14 L15 | L16 L17 L18 L19 | S11 L20 L21 S12 S13 S14 S15 S16 S17 S18 S19 S20 L22 L23 S21 S22 S23 S24 S25 S26 S27 | S28 L24 L25 S29 S30 S31 S32 S33 S34 S35 S36 S37 L26 L27 S38 S39 S40 S41 S42 S43 S44 | S45 S46 S47 S48 L28 L29 S49 S50 S51 L30 L31 S52 S53 | S58 S59 S60 S61 S62 L33 L34 S63 S64 S65 S66 S67 L35 L36 S68 S69 | S70 L37 L38 L39 L40 L41 L42 L43 L44 L45 L46 L47 S71 S72 S73 L48 L49 S74 | L50 L51 L52 L53 | L54 L55 L56 L57 | S75 S76 S77 S78 | L58 L59 S83 S84 S85 L60 L61 L62 L63 L64 S86 S87 L65 | L76 L77 L78 L79 | S96 S97 S98 S99 S100 S101 L80 S102 S103 S104 L81 L82 S105 S106 S107 L83 L84 L85 | S112 L87 L88 L89 L90 L91 L92 L93 L94 L95 L96 L97 S113 S114 S115 L98 L99 S116 | L100 S117 S118 L101 L102 L103 L104 L105 L106 L107 L108 L109 L110 L111 S119 S120 L112 | S121 S122 S123 S124 | L113 S129 S130 L114 L115 L116 L117 L118 S131 S132 L119 | L120 S133 S134 S135 S136 L121 L122 L123 S137 S138 S139 L124 L125 L126 L127 L128 S140 S141 S142 S143 S144 L129 L130 | L131 L132 L133 L134 | L135 S145 S146 S147 S148 L136 L137 L138 S149 S150 S151 L139 L140 L141 L142 L143 S152 S153 S154 S155 S156 L144 L145 | L146 S157 S158 S159 S160 L147 L148 L149 S161 S162 S163 L150 L151 L152 L153 L154 S164 S165 S166 S167 S168 L155 L156 | L157 L158 L159 L160 | L161 L162 L163 L164 L165 L166 L167 | L168 L169 L170 L171 L172 L173 S169 L174 L175 L176 L177 picked at (-3.0095, 17.219)
body "Solid1"
